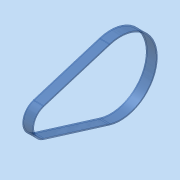
# Autodesk Inventor part: TimingBlet
Saved by Autodesk Inventor 2015 SP1 (Build 190203100, 203)
## iProperties
Created: 2015-06-16
Part Number: TimingBlet
Material: Rubber
Document SubType Name: Modeling
Designer: YOUR_NAME_HERE
Density: 0.93 g/cm^3
Appearance: Tropical Blue
Author: YOUR_NAME_HERE
Autodesk Inventor part; units mm, degrees
ref_plane "YZ Plane" through (0, 0, 0) normal (1, 0, 0) x (0, 1, 0)
ref_plane "XZ Plane" through (0, 0, 0) normal (0, 1, 0) x (-1, 0, 0)
ref_plane "XY Plane" through (0, 0, 0) normal (0, 0, 1) x (1, 0, 0)
sketch "Sketch2" plane through (0, 0, 0) normal (1, 0, 0) x (0, 1, 0)
  circle A0 centre (0, 0) radius 31.85 construction
  circle A1 centre (0, 64.66) radius 12.75 construction
  line L0 (12.181, 68.4262) -> (30.4287, 9.4082)
  line L1 (-12.181, 68.4262) -> (-30.4287, 9.4082)
  arc A2 (12.181, 68.4262) -> (-12.181, 68.4262) centre (0, 64.66) ccw
  arc A3 (-30.4287, 9.4082) -> (30.4287, 9.4082) centre (0, 0) ccw
  line L2 (31.5179, 9.745) -> (13.2702, 68.763)
  arc A4 (13.2702, 68.763) -> (-13.2702, 68.763) centre (0, 64.66) ccw
  line L3 (-13.2702, 68.763) -> (-31.5179, 9.745)
  arc A5 (-31.5179, 9.745) -> (31.5179, 9.745) centre (0, 0) ccw
  dimension "d0" = 63.7
  dimension "d1" = 25.5
  dimension "d2" = 64.66
  dimension "d3" = 1.14
  constraints: 12 point on circle, 8 end point, 6 centre point, 4 tangent, 3 coincident, 1 vertical alignment, 3 other
  measures "d0" diameter of A0
  measures "d1" diameter of A1
  measures "d2" distance of point (0, 0) A1.centre
  measures "d3" distance between parallel lines of L2 L0
extrude "Extrusion1" add sketch "Sketch2" along normal mid plane 9
body "Solid1"
